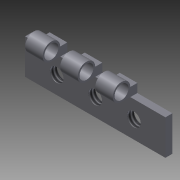
# Autodesk Inventor part: HingeP2
Saved by Autodesk Inventor 2012 (Build 160160000, 160)
## iProperties
Created: 2011-10-18
Part Number: HingeP2
Material: Default
Document SubType Name: Modeling
Designer: Smeet
Density: 1 g/cm^3
Author: Smeet
Autodesk Inventor part; units mm, degrees
ref_plane "YZ Plane" through (0, 0, 0) normal (1, 0, 0) x (0, 1, 0)
ref_plane "XZ Plane" through (0, 0, 0) normal (0, 1, 0) x (-1, 0, 0)
sketch "Sketch1" plane through (0, 0, 0) normal (0, 0, 1) x (1, 0, 0)
  line L0 (-28.3759, 9.1241) -> (22.4241, 9.1241)
  line L1 (22.4241, 9.1241) -> (22.4241, -3.5759)
  line L2 (22.4241, -3.5759) -> (-28.3759, -3.5759)
  line L3 (-28.3759, -3.5759) -> (-28.3759, 9.1241)
  point P0 (0, 0)
  dimension "d0" = 50.8
  dimension "d1" = 12.7
  constraints: 8 end point, 2 parallel, 1 horizontal, 1 perpendicular
  measures "d0" distance of L0.start L0.end
  measures "d1" distance of L2.end L0.start
extrude "Extrusion1" add sketch "Sketch1" along normal blind 2.54
sketch "Sketch2" plane through (22.4241, -3.5759, 0) normal (1, 0, 0) x (0, 0, -1)
  line L0 (0, 12.7) -> (6.35, 12.7)
  line L1 (6.35, 12.7) -> (6.35, 19.05)
  line L2 (6.35, 19.05) -> (0, 19.05)
  line L3 (0, 19.05) -> (0, 12.7)
  line L4 (0, 0) -> (-2.54, 0) projected
  line L5 (0, 12.7) -> (-2.54, 12.7) projected
  line L6 (-1.27, 12.7) -> (-1.27, 0)
  line L7 (-2.54, 12.7) -> (-8.89, 12.7)
  line L8 (-8.89, 12.7) -> (-8.89, 19.05)
  line L9 (-8.89, 19.05) -> (-2.54, 19.05)
  line L10 (-2.54, 19.05) -> (-2.54, 12.7)
  point P0 (0, 3.5759)
  dimension "d4" = 6.35
  dimension "d5" = 6.35
  constraints: 18 end point, 3 symmetric about line, 2 midpoint, 2 parallel, 1 horizontal, 1 perpendicular
  measures "d4" distance of L1.end L2.end
  measures "d5" distance of L0.end L1.end
ref_plane "Work Plane2" through (-28.3759, 9.1241, 0) normal (0, 0, 1) x (1, 0, 0)
sketch "Sketch3" plane through (-28.3759, 9.1241, 0) normal (0, 0, 1) x (1, 0, 0)
  line L0 (38.1, 0) -> (31.75, 0)
  line L1 (31.75, 0) -> (31.75, 7.3179)
  line L2 (31.75, 7.3179) -> (38.1, 7.3179)
  line L3 (38.1, 7.3179) -> (38.1, 0)
  line L4 (25.4, 0) -> (19.05, 0)
  line L5 (19.05, 0) -> (19.05, 7.3179)
  line L6 (19.05, 7.3179) -> (25.4, 7.3179)
  line L7 (25.4, 7.3179) -> (25.4, 0)
  line L8 (12.7, 0) -> (6.35, 0)
  line L9 (6.35, 0) -> (6.35, 7.3179)
  line L10 (6.35, 7.3179) -> (12.7, 7.3179)
  line L11 (12.7, 7.3179) -> (12.7, 0)
  line L12 (38.1, 7.3179) -> (50.8, 7.3179)
  line L13 (38.1, 0) -> (38.1, 7.3179)
  line L14 (25.4, 7.3179) -> (31.75, 7.3179)
  line L15 (31.75, 7.3179) -> (31.75, 0)
  line L16 (31.75, 0) -> (25.4, 0)
  line L17 (25.4, 0) -> (25.4, 7.3179)
  line L18 (12.7, 7.3179) -> (19.05, 7.3179)
  line L19 (19.05, 7.3179) -> (19.05, 0)
  line L20 (19.05, 0) -> (12.7, 0)
  line L21 (12.7, 0) -> (12.7, 7.3179)
  line L22 (6.35, 0) -> (0, 0)
  line L23 (0, 0) -> (0, 7.3179)
  line L24 (0, 7.3179) -> (6.35, 7.3179)
  line L25 (6.35, 7.3179) -> (6.35, 0)
  line L26 (50.8, 7.3179) -> (50.8, 0)
  line L27 (50.8, 0) -> (38.1, 0)
  point P0 (28.3759, -9.1241)
  constraints: 56 end point, 13 parallel, 7 horizontal, 7 perpendicular
extrude "Extrusion4" add sketch "Sketch2" against normal blind 50.8 contours L7 L8 L9 L10
fillet "Fillet2" radius 3.175 3 edges at (-2.9759, 15.4741, 8.89) (-2.9759, 15.4741, 2.54) (-2.9759, 9.1241, 8.89)
extrude "Extrusion5" cut sketch "Sketch3" along normal blind 50.8 contours L3 L12 L26 L27 | L16 L7 L14 L1 | L20 L11 L18 L5 | L22 L23 L24 L9
hole "Hole3" at (9.7241, 12.2991, 5.715) direction (-1, 0, 0) diameter 5.08 end through all
hole "Hole4" at (-16.9459, 2.7741, 2.54) direction (0, 0, -1) diameter 4.9784 end through all thread size "1/4-20 UNC" class "2B" standard "ANSI Unified Screw Threads"
hole "Hole5" at (10.9941, 2.7741, 2.54) direction (0, 0, -1) diameter 4.9784 end through all thread size "1/4-20 UNC" class "2B" standard "ANSI Unified Screw Threads"
hole "Hole6" at (-2.9759, 2.7741, 2.54) direction (0, 0, -1) diameter 4.9784 end through all thread size "1/4-20 UNC" class "2B" standard "ANSI Unified Screw Threads"
sketch "Sketch4" plane through (9.7241, 9.1241, 2.54) normal (0, 0, -1) x (-1, 0, 0)
  line L0 (0, 3.175) -> (0, 0) projected
  line L1 (6.35, 0) -> (0, 0) projected
  line L2 (0, 3.175) -> (6.35, 3.175)
  line L3 (6.35, 3.175) -> (6.35, 0)
  line L4 (6.35, 0) -> (0, 0)
  line L5 (0, 0) -> (0, 3.175)
  point P0 (9.7241, -9.1241)
  constraints: 8 end point, 2 parallel, 1 horizontal, 1 perpendicular
sketch "Sketch5" plane through (-2.9759, 9.1241, 2.54) normal (0, 0, -1) x (-1, 0, 0)
  line L0 (0, 3.175) -> (0, 0) projected
  line L1 (6.35, 0) -> (0, 0) projected
  line L2 (0, 3.175) -> (6.35, 3.175)
  line L3 (6.35, 3.175) -> (6.35, 0)
  line L4 (6.35, 0) -> (0, 0)
  line L5 (0, 0) -> (0, 3.175)
  point P0 (-2.9759, -9.1241)
  constraints: 8 end point, 2 parallel, 1 horizontal, 1 perpendicular
sketch "Sketch6" plane through (-15.6759, 12.2991, 2.54) normal (0, 0, -1) x (-1, 0, 0)
  line L0 (6.35, -3.175) -> (6.35, 0) projected
  line L1 (0, 0) -> (6.35, 0) projected
  line L2 (0, 0) -> (6.35, 0)
  line L3 (6.35, 0) -> (6.35, -3.175)
  line L4 (6.35, -3.175) -> (0, -3.175)
  line L5 (0, -3.175) -> (0, 0)
  point P0 (-15.6759, -12.2991)
  constraints: 8 end point, 2 parallel, 1 horizontal, 1 perpendicular
extrude "Extrusion6" add sketch "Sketch4" along normal blind 2.54
extrude "Extrusion7" add sketch "Sketch5" along normal blind 2.54
extrude "Extrusion8" add sketch "Sketch6" along normal blind 2.54
body "Solid1"
